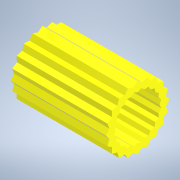
# Autodesk Inventor part: FlexRoller
Saved by Autodesk Inventor 2021 (Build 250183000, 183)
## iProperties
Created: 2021-05-21
Part Number: FlexRoller
Material: PC/ABS Plastic
Document SubType Name: Modeling
Designer: sami8
Density: 0.357273 g/cm^3
Appearance: Smooth - Yellow
Author: sami8
Autodesk Inventor part; units mm, degrees
ref_plane "YZ Plane" through (0, 0, 0) normal (1, 0, 0) x (0, 1, 0)
ref_plane "XZ Plane" through (0, 0, 0) normal (0, 1, 0) x (-1, 0, 0)
ref_plane "XY Plane" through (0, 0, 0) normal (0, 0, 1) x (1, 0, 0)
sketch "Sketch2" plane through (0, 0, 0) normal (1, 0, 0) x (0, 1, 0)
  circle A0 centre (0, 0) radius 15 construction
  circle A1 centre (0, 0) radius 18 construction
  line L0 (17.7784, 2.8158) -> (17.7784, -2.8158) construction
  line L1 (17.7784, 2.8158) -> (0, 0) construction
  line L2 (0, 0) -> (17.7784, -2.8158) construction
  line L3 (17.7784, 2.8158) -> (19.9784, 0)
  line L4 (19.9784, 0) -> (17.7784, -2.8158)
  line L5 (19.9784, 0) -> (17.7784, 0) construction
  line L6 (14.8153, 2.3465) -> (13.8153, 0)
  line L7 (13.8153, 0) -> (14.8153, -2.3465)
  line L8 (14.8153, 2.3465) -> (14.8153, -2.3465) construction
  line L9 (13.8153, 0) -> (14.8153, 0) construction
  line L10 (16.0381, 8.1718) -> (19.0006, 6.1737)
  line L11 (19.0006, 6.1737) -> (17.7784, 2.8158)
  line L12 (13.3651, 6.8099) -> (13.1392, 4.2692)
  line L13 (13.1392, 4.2692) -> (14.8153, 2.3465)
  line L14 (12.7279, 12.7279) -> (16.1629, 11.743)
  line L15 (16.1629, 11.743) -> (16.0381, 8.1718)
  line L16 (10.6066, 10.6066) -> (11.1768, 8.1204)
  line L17 (11.1768, 8.1204) -> (13.3651, 6.8099)
  line L18 (8.1718, 16.0381) -> (11.743, 16.1629)
  line L19 (11.743, 16.1629) -> (12.7279, 12.7279)
  line L20 (6.8099, 13.3651) -> (8.1204, 11.1768)
  line L21 (8.1204, 11.1768) -> (10.6066, 10.6066)
  line L22 (2.8158, 17.7784) -> (6.1737, 19.0006)
  line L23 (6.1737, 19.0006) -> (8.1718, 16.0381)
  line L24 (2.3465, 14.8153) -> (4.2692, 13.1392)
  line L25 (4.2692, 13.1392) -> (6.8099, 13.3651)
  line L26 (-2.8158, 17.7784) -> (0, 19.9784)
  line L27 (0, 19.9784) -> (2.8158, 17.7784)
  line L28 (-2.3465, 14.8153) -> (0, 13.8153)
  line L29 (0, 13.8153) -> (2.3465, 14.8153)
  line L30 (-8.1718, 16.0381) -> (-6.1737, 19.0006)
  line L31 (-6.1737, 19.0006) -> (-2.8158, 17.7784)
  line L32 (-6.8099, 13.3651) -> (-4.2692, 13.1392)
  line L33 (-4.2692, 13.1392) -> (-2.3465, 14.8153)
  line L34 (-12.7279, 12.7279) -> (-11.743, 16.1629)
  line L35 (-11.743, 16.1629) -> (-8.1718, 16.0381)
  line L36 (-10.6066, 10.6066) -> (-8.1204, 11.1768)
  line L37 (-8.1204, 11.1768) -> (-6.8099, 13.3651)
  line L38 (-16.0381, 8.1718) -> (-16.1629, 11.743)
  line L39 (-16.1629, 11.743) -> (-12.7279, 12.7279)
  line L40 (-13.3651, 6.8099) -> (-11.1768, 8.1204)
  line L41 (-11.1768, 8.1204) -> (-10.6066, 10.6066)
  line L42 (-17.7784, 2.8158) -> (-19.0006, 6.1737)
  line L43 (-19.0006, 6.1737) -> (-16.0381, 8.1718)
  line L44 (-14.8153, 2.3465) -> (-13.1392, 4.2692)
  line L45 (-13.1392, 4.2692) -> (-13.3651, 6.8099)
  line L46 (-17.7784, -2.8158) -> (-19.9784, 0)
  line L47 (-19.9784, 0) -> (-17.7784, 2.8158)
  line L48 (-14.8153, -2.3465) -> (-13.8153, 0)
  line L49 (-13.8153, 0) -> (-14.8153, 2.3465)
  line L50 (-16.0381, -8.1718) -> (-19.0006, -6.1737)
  line L51 (-19.0006, -6.1737) -> (-17.7784, -2.8158)
  line L52 (-13.3651, -6.8099) -> (-13.1392, -4.2692)
  line L53 (-13.1392, -4.2692) -> (-14.8153, -2.3465)
  line L54 (-12.7279, -12.7279) -> (-16.1629, -11.743)
  line L55 (-16.1629, -11.743) -> (-16.0381, -8.1718)
  line L56 (-10.6066, -10.6066) -> (-11.1768, -8.1204)
  line L57 (-11.1768, -8.1204) -> (-13.3651, -6.8099)
  line L58 (-8.1718, -16.0381) -> (-11.743, -16.1629)
  line L59 (-11.743, -16.1629) -> (-12.7279, -12.7279)
  line L60 (-6.8099, -13.3651) -> (-8.1204, -11.1768)
  line L61 (-8.1204, -11.1768) -> (-10.6066, -10.6066)
  line L62 (-2.8158, -17.7784) -> (-6.1737, -19.0006)
  line L63 (-6.1737, -19.0006) -> (-8.1718, -16.0381)
  line L64 (-2.3465, -14.8153) -> (-4.2692, -13.1392)
  line L65 (-4.2692, -13.1392) -> (-6.8099, -13.3651)
  line L66 (2.8158, -17.7784) -> (0, -19.9784)
  line L67 (0, -19.9784) -> (-2.8158, -17.7784)
  line L68 (2.3465, -14.8153) -> (0, -13.8153)
  line L69 (0, -13.8153) -> (-2.3465, -14.8153)
  line L70 (8.1718, -16.0381) -> (6.1737, -19.0006)
  line L71 (6.1737, -19.0006) -> (2.8158, -17.7784)
  line L72 (6.8099, -13.3651) -> (4.2692, -13.1392)
  line L73 (4.2692, -13.1392) -> (2.3465, -14.8153)
  line L74 (12.7279, -12.7279) -> (11.743, -16.1629)
  line L75 (11.743, -16.1629) -> (8.1718, -16.0381)
  line L76 (10.6066, -10.6066) -> (8.1204, -11.1768)
  line L77 (8.1204, -11.1768) -> (6.8099, -13.3651)
  line L78 (16.0381, -8.1718) -> (16.1629, -11.743)
  line L79 (16.1629, -11.743) -> (12.7279, -12.7279)
  line L80 (13.3651, -6.8099) -> (11.1768, -8.1204)
  line L81 (11.1768, -8.1204) -> (10.6066, -10.6066)
  line L82 (17.7784, -2.8158) -> (19.0006, -6.1737)
  line L83 (19.0006, -6.1737) -> (16.0381, -8.1718)
  line L84 (14.8153, -2.3465) -> (13.1392, -4.2692)
  line L85 (13.1392, -4.2692) -> (13.3651, -6.8099)
  dimension "d15" = 30
  dimension "d16" = 36
  dimension "d19" = 18
  dimension "d20" = 2.2
  dimension "d22" = 1
  dimension "d25" = 360
  constraints: 172 end point, 4 point on circle, 3 coincident, 2 centre point, 2 horizontal, 2 midpoint, 2 point on line, 2 vertical, 201 other
  measures "d15" diameter of A0
  measures "d16" diameter of A1
  measures "d19" angle of L1 L2
  measures "d20" distance of L4.start L5.end
  measures "d22" distance from line of L8 L6.end
extrude "Extrusion2" add sketch "Sketch2" along normal blind 60
body "Solid2"
